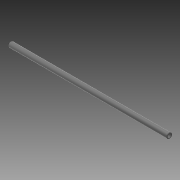
# Autodesk Inventor part: CF Tube 8x10x250
Saved by Autodesk Inventor 2020 (Build 240168000, 168)
## iProperties
Created: 2021-05-05
Part Number: CF Tube 8x10x250
Material: Generic
Document SubType Name: Modeling
Designer: DDeGo
Density: 1 g/cm^3
Appearance: Default
Author: DDeGo
Autodesk Inventor part; units mm, degrees
ref_plane "YZ Plane" through (0, 0, 0) normal (1, 0, 0) x (0, 1, 0)
ref_plane "XZ Plane" through (0, 0, 0) normal (0, 1, 0) x (-1, 0, 0)
ref_plane "XY Plane" through (0, 0, 0) normal (0, 0, 1) x (1, 0, 0)
sketch "Sketch1" plane through (0, 0, 0) normal (0, 0, 1) x (1, 0, 0)
  line L0 (0, 3) -> (-250, 3)
  line L1 (-250, 3) -> (-250, 4)
  line L2 (-250, 4) -> (0, 4)
  line L3 (0, 4) -> (0, 3)
  line L4 (0, 3) -> (0, 0) construction
  line L5 (0, 0) -> (-250, 0) construction
  line L6 (-250, 0) -> (-250, 3) construction
  dimension "d0" = 3
  dimension "d1" = 4
  dimension "d2" = 250
  constraints: 14 end point, 2 parallel, 2 perpendicular, 1 collinear, 1 horizontal, 1 vertical
  measures "d0" distance between parallel lines of L5 L0
  measures "d1" distance between parallel lines of L5 L2
  measures "d2" distance of L4.end L5.end
revolve "Revolution1" add sketch "Sketch1" angle 360 about axis through (0, 0, 0) along (-1, 0, 0)
chamfer "Chamfer1" distance 0.5 angle 45 2 edges at (0, -4, 0) (-250, -4, 0)
body "Solid1"
